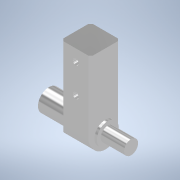
# Autodesk Inventor part: Brazo
Saved by Autodesk Inventor 2022 (Build 260153000, 153)
## iProperties
Created: 2021-10-22
Part Number: Brazo
Material: Aluminum 6061
Document SubType Name: Modeling
Designer: juanp
Density: 2.7 g/cm^3
Appearance: Aluminum - Flat
Author: juanp
Autodesk Inventor part; units mm, degrees
ref_plane "YZ Plane" through (0, 0, 0) normal (1, 0, 0) x (0, 1, 0)
ref_plane "XZ Plane" through (0, 0, 0) normal (0, 1, 0) x (-1, 0, 0)
sketch "Sketch1" plane through (0, 0, 0) normal (0, 1, 0) x (-1, 0, 0)
  line L0 (13.7, 13.7) -> (-13.7, 13.7)
  line L1 (-13.7, 13.7) -> (-13.7, -13.7)
  line L2 (-13.7, -13.7) -> (13.7, -13.7)
  line L3 (13.7, -13.7) -> (13.7, 13.7)
  line L4 (13.7, 13.7) -> (-13.7, -13.7) construction
  line L5 (-13.7, 13.7) -> (13.7, -13.7) construction
  line L6 (-12.7, -12.7) -> (12.7, -12.7)
  line L7 (12.7, -12.7) -> (12.7, 12.7)
  line L8 (12.7, 12.7) -> (-12.7, 12.7)
  line L9 (-12.7, 12.7) -> (-12.7, -12.7)
  line L10 (-12.7, -12.7) -> (12.7, 12.7) construction
  line L11 (12.7, -12.7) -> (-12.7, 12.7) construction
  point P0 (0, 0)
  dimension "d1" = 1
  dimension "d35" = 25.4
  constraints: 24 end point, 4 midpoint, 4 parallel, 3 perpendicular, 2 horizontal, 1 point on line
  measures "d1" distance between parallel lines of L3 L7
  measures "d35" distance between parallel lines of L6 L8
extrude "Extrusion1" add sketch "Sketch1" along normal blind 417.154
fillet "Fillet1" radius 2 8 edges at (-12.7, 208.577, 12.7) (13.7, 208.577, -13.7) (-13.7, 208.577, -13.7) (12.7, 208.577, -12.7) (-12.7, 208.577, -12.7) (12.7, 208.577, 12.7) (13.7, 208.577, 13.7) (-13.7, 208.577, 13.7)
ref_plane "Work Plane1" through (-13.7, 417.154, 13.7) normal (0, 0.7504226, 0.6609583) x (1, 0, 0)
sketch "Sketch4" plane through (0, 0, 0) normal (0, -1, 0) x (1, 0, 0)
  line L0 (12.7, -12.7) -> (-12.7, -12.7)
  line L1 (-12.7, -12.7) -> (-12.7, 12.7)
  line L2 (-12.7, 12.7) -> (12.7, 12.7)
  line L3 (12.7, 12.7) -> (12.7, -12.7)
  line L4 (12.7, -12.7) -> (-12.7, 12.7) construction
  line L5 (-12.7, -12.7) -> (12.7, 12.7) construction
  line L6 (12.7, 12.7) -> (-12.7, 12.7) projected
  point P0 (0, 0)
  dimension "d9" = 0
  constraints: 12 end point, 2 midpoint, 2 parallel, 2 perpendicular, 1 horizontal
  measures "d9" distance between parallel lines of L6 L2
extrude "Extrusion3" add sketch "Sketch4" against normal blind 75 separate body
sketch "Sketch6" plane through (0, 0, 0) normal (0, -1, 0) x (1, 0, 0)
  line L0 (13.7, 11.7) -> (13.7, -11.7) projected
  line L1 (-11.7, 13.7) -> (11.7, 13.7) projected
  line L2 (-13.7, -11.7) -> (-13.7, 11.7) projected
  line L3 (11.7, -13.7) -> (-11.7, -13.7) projected
  line L4 (12.7, -10.7) -> (12.7, 10.7) projected
  line L5 (-10.7, -12.7) -> (10.7, -12.7) projected
  line L6 (-12.7, 10.7) -> (-12.7, -10.7) projected
  line L7 (10.7, 12.7) -> (-10.7, 12.7) projected
  arc A0 (-11.7, 13.7) -> (-13.7, 11.7) centre (-11.7, 11.7) ccw projected
  arc A1 (-13.7, -11.7) -> (-11.7, -13.7) centre (-11.7, -11.7) ccw projected
  arc A2 (11.7, -13.7) -> (13.7, -11.7) centre (11.7, -11.7) ccw projected
  arc A3 (13.7, 11.7) -> (11.7, 13.7) centre (11.7, 11.7) ccw projected
  arc A4 (10.7, -12.7) -> (12.7, -10.7) centre (10.7, -10.7) ccw projected
  arc A5 (-12.7, -10.7) -> (-10.7, -12.7) centre (-10.7, -10.7) ccw projected
  arc A6 (-10.7, 12.7) -> (-12.7, 10.7) centre (-10.7, 10.7) ccw projected
  arc A7 (12.7, 10.7) -> (10.7, 12.7) centre (10.7, 10.7) ccw projected
  point P0 (0, 0)
extrude "Extrusion5" cut sketch "Sketch6" against normal blind 30 contours L0 A2 L3 A1 L2 A0 L1 A3 | A4 L5 A5 L6 A6 L7 A7 L4 bodies 1
sketch "Sketch7" plane through (-13.7, 417.154, 13.7) normal (0, 0, 1) x (1, 0, 0)
  line L0 (13.7, -377.154) -> (13.7, -352.154) construction
  line L1 (13.7, -352.154) -> (13.7, -342.154) construction
  line L2 (13.7, -377.154) -> (13.7, -387.154) construction
  circle A0 centre (13.7, -352.154) radius 2.55
  circle A1 centre (13.7, -377.154) radius 2.55
  line L3 (1, -342.154) -> (26.4, -342.154) projected
  line L4 (2, -387.154) -> (25.4, -387.154) projected
  point P0 (0, -299.6)
  point P1 (27.4, -299.6)
  dimension "d20" = 5.1
  dimension "d21" = 10
  constraints: 7 end point, 2 centre point, 2 coincident, 2 collinear, 1 equal radius, 1 midpoint, 1 vertical, 2 other
  measures "d20" diameter of A1
  measures "d21" distance of L1.end L0.end
extrude "Extrusion6" cut sketch "Sketch7" against normal through all bodies 1 2
sketch "Sketch8" plane through (-13.7, 417.154, 13.7) normal (0, 0, 1) x (1, 0, 0)
  line L0 (27.4, 0) -> (0, 0) projected
  line L1 (13.7, 0) -> (13.7, -7.5) construction
  line L2 (13.7, -7.5) -> (13.7, -32.5) construction
  circle A0 centre (13.7, -7.5) radius 2.65
  circle A1 centre (13.7, -32.5) radius 2.65
  point P0 (13.7, -417.154)
  point P1 (27.4, -299.6)
  point P2 (0, -299.6)
  dimension "d26" = 7.5
  dimension "d27" = 25
  dimension "d28" = 5.3
  dimension "d29" = 5.3
  constraints: 4 end point, 2 centre point, 2 coincident, 1 midpoint, 1 point on line, 1 vertical
  measures "d26" distance of L1.start L1.end
  measures "d27" distance of L1.end L2.end
  measures "d28" diameter of A0
  measures "d29" diameter of A1
extrude "Extrusion7" cut sketch "Sketch8" against normal through all bodies 1
sketch "Sketch13" plane through (-12.7, 0, -12.7) normal (-1, 0, 0) x (0, 0, 1)
  line L0 (0, 0) -> (0, 75) projected
  line L1 (25.4, 0) -> (0, 0) projected
  line L2 (25.4, 0) -> (25.4, 75) projected
  circle A0 centre (12.7, 12.7) radius 6 construction
  circle A1 centre (12.7, 12.7) radius 9.35
  circle A2 centre (12.7, 12.7) radius 12.7
  line L3 (12.7, 12.7) -> (6.7, 12.7) construction
  line L4 (3.35, 12.7) -> (0, 12.7) construction
  line L5 (0, 0) -> (0, 75) projected
  line L6 (3.35, 12.7) -> (6.7, 12.7) construction
  point P0 (12.7, 0)
  point P1 (6.1952, 0)
  point P2 (25.4, 12.7)
  point P3 (12.7, 0)
  point P4 (5.5838, 6.6351)
  point P5 (19.8162, 6.6351)
  point P6 (19.8162, 18.7649)
  point P7 (5.5838, 18.7649)
  dimension "d58" = 12
  dimension "d68" = 3.35
  constraints: 6 end point, 5 point on circle, 3 horizontal, 2 coincident, 2 point on line, 2 vertical, 1 centre point, 1 collinear, 1 horizontal alignment, 5 other
  measures "d68" distance of L4.start L4.end
extrude "Extrusion14" cut sketch "Sketch13" against normal through all contours L0 A2 L1 | A2 L2 L1 | A1 bodies 2
extrude "Extrusion15" add sketch "Sketch13" against normal up to surface (25.4 mm away) separate body contours A1
sketch "Sketch15" plane through (-12.7, 0, -12.7) normal (-1, 0, 0) x (0, 0, 1)
  circle A0 centre (12.7, 12.7) radius 9.35 projected
  circle A1 centre (12.7, 12.7) radius 9.35
  circle A2 centre (12.7, 12.7) radius 6
  point P0 (12.7, 0)
  point P1 (19.5401, 6.5)
  point P2 (22.05, 12.7)
  dimension "d70" = 12
  constraints: 2 centre point, 2 coincident, 1 concentric
  measures "d70" diameter of A2
extrude "Extrusion16" add sketch "Sketch15" along normal blind 23 bodies 3
sketch "Sketch16" plane through (-12.7, 12.7, 0) normal (-1, 0, 0) x (0, 0, 1)
  circle A0 centre (0, 0) radius 6 projected
  point P0 (0, -12.7)
extrude "Extrusion17" add sketch "Sketch16" along normal blind 3 bodies 3
sketch "Sketch19" plane through (12.7, 12.7, 0) normal (1, 0, 0) x (0, -1, 0)
  circle A0 centre (0, 0) radius 9.35 projected
  point P0 (12.7, 0)
extrude "Extrusion20" add sketch "Sketch19" along normal blind 2 bodies 3
sketch "Sketch17" plane through (14.7, 12.7, 0) normal (1, 0, 0) x (0, 0, -1)
  circle A0 centre (0, 0) radius 6
  point P0 (0, -12.7)
  dimension "d75" = 12
  constraints: 1 centre point, 1 coincident
  measures "d75" diameter of A0
extrude "Extrusion18" add sketch "Sketch17" along normal blind 20 bodies 3
sketch "Sketch18" plane through (-35.7, 12.7, 0) normal (-1, 0, 0) x (0, 0, 1)
  circle A0 centre (0, 0) radius 6 projected
  line L0 (-2, -5.6569) -> (2, -5.6569)
  line L1 (2, -5.6569) -> (2, -8)
  line L2 (2, -8) -> (-2, -8)
  line L3 (-2, -8) -> (-2, -5.6569)
  line L4 (0, -5.6569) -> (0, -6) construction
  point P0 (0, -12.7)
  point P1 (-1.94, -6.1429)
  point P2 (-1.94, -6.1429)
  dimension "d85" = 4
  dimension "d97" = 2
  constraints: 10 end point, 3 point on circle, 2 parallel, 1 coincident, 1 horizontal, 1 line through centre, 1 midpoint, 1 perpendicular, 1 vertical, 2 other
  measures "d85" distance of L0.start L0.end
  measures "d97" distance from line of L2 L4.end
extrude "Extrusion19" cut sketch "Sketch18" against normal up to surface (20 mm away) contours L0 A0 | A0 L1 L2 L3 picked at (-0.2261, -5.7584) bodies 3
chamfer "Chamfer1" distance 2 angle 45 4 edges at (12.7, 43.85, 12.7) (-12.7, 43.85, 12.7) (12.7, 43.85, -12.7) (-12.7, 43.85, -12.7)
body "Solid1"
body "Solid2"
body "Solid6"
